Autodesk Inventor part; units mm, degrees
(part 3 of 4)
sketch "Эскиз41" plane through (1.5, 0, 0) normal (1, 0, 0) x (0, 0, -1)
  circle A0 centre (383.6, 368.9) radius 1.625 projected
  circle A1 centre (-13.6, 369) radius 1.625 projected
  circle A2 centre (383.6, 1.1) radius 1.625 projected
  circle A3 centre (-13.6, 1.1) radius 1.625 projected
  circle A4 centre (379.0468, 185.0848) radius 1.625 projected
  circle A5 centre (-9.0468, 185.0848) radius 1.625 projected
  circle A6 centre (379, 228) radius 1.625 projected
  circle A7 centre (-9, 228) radius 1.625 projected
  circle A8 centre (316, 368) radius 1.625 projected
  circle A9 centre (299, 228) radius 1.625 projected
  circle A10 centre (54, 228) radius 1.625 projected
  circle A11 centre (71, 142) radius 1.625 projected
  circle A12 centre (71, 2.0002) radius 1.625 projected
  circle A13 centre (54, 2.0002) radius 1.625 projected
  circle A14 centre (71, 368) radius 1.625 projected
  circle A15 centre (71, 228) radius 1.625 projected
  circle A16 centre (316, 142) radius 1.625 projected
  circle A17 centre (316, 228) radius 1.625 projected
  circle A18 centre (183.175, 129.0059) radius 1.85 projected
  circle A19 centre (299, 368) radius 1.625 projected
  circle A20 centre (316, 2.0002) radius 1.625 projected
  circle A21 centre (54, 142) radius 1.625 projected
  circle A22 centre (54, 368) radius 1.625 projected
  circle A23 centre (299, 2.0002) radius 1.625 projected
  circle A24 centre (299, 142) radius 1.625 projected
  arc A25 (185, 193.309) -> (185, 192.7028) centre (183.175, 193.0059) ccw projected
  line L0 (185, 193.309) -> (185, 192.7028) projected
  line L1 (14.5, 247.5001) -> (35, 247.5001) projected
  arc A26 (38, 244.5001) -> (35, 247.5001) centre (35, 244.5001) ccw projected
  line L2 (38, 244.5001) -> (38, 185.5001) projected
  arc A27 (35, 182.5001) -> (38, 185.5001) centre (35, 185.5001) ccw projected
  line L3 (35, 182.5001) -> (14.5, 182.5001) projected
  arc A28 (11.5, 185.5001) -> (14.5, 182.5001) centre (14.5, 185.5001) ccw projected
  line L4 (11.5, 185.5001) -> (11.5, 244.5001) projected
  arc A29 (14.5, 247.5001) -> (11.5, 244.5001) centre (14.5, 244.5001) ccw projected
  line L5 (358.5, 244.5001) -> (358.5, 185.5001) projected
  arc A30 (355.5, 182.5001) -> (358.5, 185.5001) centre (355.5, 185.5001) ccw projected
  line L6 (355.5, 182.5001) -> (335, 182.5001) projected
  arc A31 (332, 185.5001) -> (335, 182.5001) centre (335, 185.5001) ccw projected
  line L7 (332, 185.5001) -> (332, 244.5001) projected
  arc A32 (335, 247.5001) -> (332, 244.5001) centre (335, 244.5001) ccw projected
  line L8 (335, 247.5001) -> (355.5, 247.5001) projected
  arc A33 (358.5, 244.5001) -> (355.5, 247.5001) centre (355.5, 244.5001) ccw projected
  line L9 (98.825, 226.3849) -> (98.825, 137.3849) projected
  arc A34 (95.825, 134.3849) -> (98.825, 137.3849) centre (95.825, 137.3849) ccw projected
  line L10 (95.825, 134.3849) -> (87.825, 134.3849) projected
  arc A35 (84.825, 137.3849) -> (87.825, 134.3849) centre (87.825, 137.3849) ccw projected
  line L11 (84.825, 137.3849) -> (84.825, 226.3849) projected
  arc A36 (87.825, 229.3849) -> (84.825, 226.3849) centre (87.825, 226.3849) ccw projected
  line L12 (87.825, 229.3849) -> (95.825, 229.3849) projected
  arc A37 (98.825, 226.3849) -> (95.825, 229.3849) centre (95.825, 226.3849) ccw projected
  circle A38 centre (124.375, 129.0059) radius 2 projected
  circle A39 centre (124.375, 193.0059) radius 2 projected
  circle A40 centre (217.25, 312.9941) radius 2.1 projected
  circle A41 centre (152.75, 57.0059) radius 2.1 projected
  circle A42 centre (152.75, 118.0059) radius 2.1 projected
  circle A43 centre (152.75, 312.9941) radius 2.1 projected
  circle A44 centre (217.25, 251.9941) radius 2.1 projected
  circle A45 centre (217.25, 57.0059) radius 2.1 projected
  circle A46 centre (217.25, 118.0059) radius 2.1 projected
  circle A47 centre (152.75, 251.9941) radius 2.1 projected
  line L13 (165, 44) -> (165, 8) projected
  arc A48 (162, 5) -> (165, 8) centre (162, 8) ccw projected
  line L14 (162, 5) -> (96, 5) projected
  arc A49 (93, 8) -> (96, 5) centre (96, 8) ccw projected
  line L15 (93, 8) -> (93, 44) projected
  arc A50 (96, 47) -> (93, 44) centre (96, 44) ccw projected
  line L16 (96, 47) -> (162, 47) projected
  arc A51 (165, 44) -> (162, 47) centre (162, 44) ccw projected
  circle A52 centre (319.1128, 165.0002) radius 2.1 projected
  circle A53 centre (287, 56.343) radius 2.1 projected
  circle A54 centre (50.8872, 165.0002) radius 2.1 projected
  circle A55 centre (173.9908, 56.343) radius 2.1 projected
  circle A56 centre (135.25, 60) radius 2.1 projected
  circle A57 centre (103, 60) radius 2.1 projected
  line L17 (226.25, 270.0041) -> (226.25, 298.657) projected
  arc A58 (228.25, 300.657) -> (226.25, 298.657) centre (228.25, 298.657) ccw projected
  line L18 (228.25, 300.657) -> (268.3252, 300.657) projected
  arc A59 (269.4885, 297.03) -> (268.3252, 300.657) centre (268.3252, 298.657) ccw projected
  line L19 (269.4885, 297.03) -> (229.4132, 268.3772) projected
  arc A60 (226.25, 270.0041) -> (229.4132, 268.3772) centre (228.25, 270.0041) ccw projected
  arc A61 (235.9248, 170.343) -> (234.7615, 166.7161) centre (235.9248, 168.343) ccw projected
  line L20 (235.9248, 170.343) -> (276, 170.343) projected
  arc A62 (278, 168.343) -> (276, 170.343) centre (276, 168.343) ccw projected
  line L21 (278, 168.343) -> (278, 139.6902) projected
  arc A63 (274.8368, 138.0633) -> (278, 139.6902) centre (276, 139.6902) ccw projected
  line L22 (274.8368, 138.0633) -> (234.7615, 166.7161) projected
  arc A64 (94, 106.343) -> (92, 104.343) centre (94, 104.343) ccw projected
  line L23 (94, 106.343) -> (134.0752, 106.343) projected
  arc A65 (135.2385, 102.7161) -> (134.0752, 106.343) centre (134.0752, 104.343) ccw projected
  line L24 (135.2385, 102.7161) -> (95.1632, 74.0633) projected
  arc A66 (92, 75.6902) -> (95.1632, 74.0633) centre (94, 75.6902) ccw projected
  line L25 (92, 75.6902) -> (92, 104.343) projected
  arc A67 (92, 265.657) -> (94, 263.657) centre (94, 265.657) ccw projected
  line L26 (92, 265.657) -> (92, 294.3098) projected
  arc A68 (95.1632, 295.9367) -> (92, 294.3098) centre (94, 294.3098) ccw projected
  line L27 (95.1632, 295.9367) -> (135.2385, 267.2839) projected
  arc A69 (134.0752, 263.657) -> (135.2385, 267.2839) centre (134.0752, 265.657) ccw projected
  line L28 (134.0752, 263.657) -> (94, 263.657) projected
  arc A70 (130.725, 206.0059) -> (132.725, 204.0059) centre (132.725, 206.0059) ccw projected
  line L29 (130.725, 206.0059) -> (130.725, 234.2716) projected
  arc A71 (133.9769, 235.8314) -> (130.725, 234.2716) centre (132.725, 234.2716) ccw projected
  line L30 (133.9769, 235.8314) -> (169.1945, 207.5656) projected
  arc A72 (167.9426, 204.0059) -> (169.1945, 207.5656) centre (167.9426, 206.0059) ccw projected
  line L31 (167.9426, 204.0059) -> (132.725, 204.0059) projected
  arc A73 (226.25, 71.343) -> (228.25, 69.343) centre (228.25, 71.343) ccw projected
  line L32 (226.25, 71.343) -> (226.25, 99.9959) projected
  arc A74 (229.4132, 101.6228) -> (226.25, 99.9959) centre (228.25, 99.9959) ccw projected
  line L33 (229.4132, 101.6228) -> (269.4885, 72.97) projected
  arc A75 (268.3252, 69.343) -> (269.4885, 72.97) centre (268.3252, 71.343) ccw projected
  line L34 (268.3252, 69.343) -> (228.25, 69.343) projected
  arc A76 (226.25, 201.657) -> (228.25, 199.657) centre (228.25, 201.657) ccw projected
  line L35 (226.25, 201.657) -> (226.25, 230.3098) projected
  arc A77 (229.4132, 231.9367) -> (226.25, 230.3098) centre (228.25, 230.3098) ccw projected
  line L36 (229.4132, 231.9367) -> (269.4885, 203.2839) projected
  arc A78 (268.3252, 199.657) -> (269.4885, 203.2839) centre (268.3252, 201.657) ccw projected
  line L37 (268.3252, 199.657) -> (228.25, 199.657) projected
  arc A79 (278, 294.3098) -> (274.8368, 295.9367) centre (276, 294.3098) ccw projected
  line L38 (278, 294.3098) -> (278, 265.657) projected
  arc A80 (276, 263.657) -> (278, 265.657) centre (276, 265.657) ccw projected
  line L39 (276, 263.657) -> (235.9248, 263.657) projected
  arc A81 (234.7615, 267.2839) -> (235.9248, 263.657) centre (235.9248, 265.657) ccw projected
  line L40 (234.7615, 267.2839) -> (274.8368, 295.9367) projected
  arc A82 (226.25, 135.343) -> (228.25, 133.343) centre (228.25, 135.343) ccw projected
  line L41 (226.25, 135.343) -> (226.25, 163.9959) projected
  arc A83 (229.4132, 165.6228) -> (226.25, 163.9959) centre (228.25, 163.9959) ccw projected
  line L42 (229.4132, 165.6228) -> (269.4885, 136.97) projected
  arc A84 (268.3252, 133.343) -> (269.4885, 136.97) centre (268.3252, 135.343) ccw projected
  line L43 (268.3252, 133.343) -> (228.25, 133.343) projected
  arc A85 (143.75, 99.9959) -> (140.5868, 101.6228) centre (141.75, 99.9959) ccw projected
  line L44 (143.75, 99.9959) -> (143.75, 71.343) projected
  arc A86 (141.75, 69.343) -> (143.75, 71.343) centre (141.75, 71.343) ccw projected
  line L45 (141.75, 69.343) -> (101.6748, 69.343) projected
  arc A87 (100.5115, 72.97) -> (101.6748, 69.343) centre (101.6748, 71.343) ccw projected
  line L46 (100.5115, 72.97) -> (140.5868, 101.6228) projected
  arc A88 (143.75, 298.657) -> (141.75, 300.657) centre (141.75, 298.657) ccw projected
  line L47 (143.75, 298.657) -> (143.75, 270.0041) projected
  arc A89 (140.5868, 268.3772) -> (143.75, 270.0041) centre (141.75, 270.0041) ccw projected
  line L48 (140.5868, 268.3772) -> (100.5115, 297.03) projected
  arc A90 (101.6748, 300.657) -> (100.5115, 297.03) centre (101.6748, 298.657) ccw projected
  line L49 (101.6748, 300.657) -> (141.75, 300.657) projected
  line L50 (176.825, 239.0059) -> (176.825, 210.7401) projected
  arc A91 (173.5731, 209.1803) -> (176.825, 210.7401) centre (174.825, 210.7401) ccw projected
  line L51 (173.5731, 209.1803) -> (138.3555, 237.4461) projected
  arc A92 (139.6074, 241.0059) -> (138.3555, 237.4461) centre (139.6074, 239.0059) ccw projected
  line L52 (139.6074, 241.0059) -> (174.825, 241.0059) projected
  arc A93 (176.825, 239.0059) -> (174.825, 241.0059) centre (174.825, 239.0059) ccw projected
  line L53 (278, 104.343) -> (278, 75.6902) projected
  arc A94 (274.8368, 74.0633) -> (278, 75.6902) centre (276, 75.6902) ccw projected
  line L54 (274.8368, 74.0633) -> (234.7615, 102.7161) projected
  arc A95 (235.9248, 106.343) -> (234.7615, 102.7161) centre (235.9248, 104.343) ccw projected
  line L55 (235.9248, 106.343) -> (276, 106.343) projected
  arc A96 (278, 104.343) -> (276, 106.343) centre (276, 104.343) ccw projected
  arc A97 (278, 234.657) -> (276, 236.657) centre (276, 234.657) ccw projected
  line L56 (278, 234.657) -> (278, 206.0041) projected
  arc A98 (274.8368, 204.3772) -> (278, 206.0041) centre (276, 206.0041) ccw projected
  line L57 (274.8368, 204.3772) -> (234.7615, 233.03) projected
  arc A99 (235.9248, 236.657) -> (234.7615, 233.03) centre (235.9248, 234.657) ccw projected
  line L58 (235.9248, 236.657) -> (276, 236.657) projected
  arc A100 (295, 375) -> (292, 372) centre (295, 372) ccw projected
  line L59 (292, 372) -> (292, 323.5966) projected
  arc A101 (289, 320.5966) -> (292, 323.5966) centre (289, 323.5966) ccw projected
  line L60 (289, 320.5966) -> (81, 320.5966) projected
  arc A102 (78, 323.5966) -> (81, 320.5966) centre (81, 323.5966) ccw projected
  line L61 (78, 323.5966) -> (78, 372) projected
  arc A103 (78, 372) -> (75, 375) centre (75, 372) ccw projected
  line L62 (75, 375) -> (-15, 375) projected
  arc A104 (-15, 375) -> (-18, 372) centre (-15, 372) ccw projected
  line L63 (-18, 372) -> (-18, -2) projected
  arc A105 (-18, -2) -> (-15, -5) centre (-15, -2) ccw projected
  line L64 (-15, -5) -> (385, -5) projected
  arc A106 (385, -5) -> (388, -2) centre (385, -2) ccw projected
  line L65 (388, -2) -> (388, 372) projected
  arc A107 (388, 372) -> (385, 375) centre (385, 372) ccw projected
  line L66 (385, 375) -> (295, 375) projected
  line L67 (49, 266.848) -> (-8, 266.848) projected
  arc A108 (-11, 269.848) -> (-8, 266.848) centre (-8, 269.848) ccw projected
  line L68 (-11, 269.848) -> (-11, 367) projected
  arc A109 (-8, 370) -> (-11, 367) centre (-8, 367) ccw projected
  line L69 (-8, 370) -> (-7.7889, 370) projected
  arc A110 (-4.2111, 370) -> (-7.7889, 370) centre (-6, 368.9) ccw projected
  line L70 (-4.2111, 370) -> (37, 370) projected
  arc A111 (40, 367) -> (37, 370) centre (37, 367) ccw projected
  line L71 (40, 367) -> (40, 341.848) projected
  arc A112 (40, 341.848) -> (43, 338.848) centre (43, 341.848) ccw projected
  line L72 (43, 338.848) -> (49, 338.848) projected
  arc A113 (52, 335.848) -> (49, 338.848) centre (49, 335.848) ccw projected
  line L73 (52, 335.848) -> (52, 269.848) projected
  arc A114 (49, 266.848) -> (52, 269.848) centre (49, 269.848) ccw projected
  line L74 (374.2111, 0) -> (333, 0) projected
  arc A115 (330, 3) -> (333, 0) centre (333, 3) ccw projected
  line L75 (330, 3) -> (330, 28.152) projected
  arc A116 (330, 28.152) -> (327, 31.152) centre (327, 28.152) ccw projected
  line L76 (327, 31.152) -> (321, 31.152) projected
  arc A117 (318, 34.152) -> (321, 31.152) centre (321, 34.152) ccw projected
  line L77 (318, 34.152) -> (318, 100.152) projected
  arc A118 (321, 103.152) -> (318, 100.152) centre (321, 100.152) ccw projected
  line L78 (321, 103.152) -> (327, 103.152) projected
  arc A119 (327, 103.152) -> (330, 106.152) centre (327, 106.152) ccw projected
  line L79 (330, 106.152) -> (330, 160) projected
  arc A120 (333, 163) -> (330, 160) centre (333, 160) ccw projected
  line L80 (333, 163) -> (377, 163) projected
  arc A121 (380, 160) -> (377, 163) centre (377, 160) ccw projected
  line L81 (380, 160) -> (380, 3) projected
  arc A122 (377.8605, 0.1261) -> (380, 3) centre (377, 3) ccw projected
  arc A123 (374.2111, 0) -> (377.8605, 0.1261) centre (376, 1.1) ccw projected
  line L82 (-7, 163) -> (37, 163) projected
  arc A124 (40, 160) -> (37, 163) centre (37, 160) ccw projected
  line L83 (40, 160) -> (40, 106.152) projected
  arc A125 (40, 106.152) -> (43, 103.152) centre (43, 106.152) ccw projected
  line L84 (43, 103.152) -> (49, 103.152) projected
  arc A126 (52, 100.152) -> (49, 103.152) centre (49, 100.152) ccw projected
  line L85 (52, 100.152) -> (52, 34.152) projected
  arc A127 (49, 31.152) -> (52, 34.152) centre (49, 34.152) ccw projected
  line L86 (49, 31.152) -> (43, 31.152) projected
  arc A128 (43, 31.152) -> (40, 28.152) centre (43, 28.152) ccw projected
  line L87 (40, 28.152) -> (40, 3) projected
  arc A129 (37, 0) -> (40, 3) centre (37, 3) ccw projected
  line L88 (37, 0) -> (-4.2111, 0) projected
  arc A130 (-7.8605, 0.1261) -> (-4.2111, 0) centre (-6, 1.1) ccw projected
  arc A131 (-10, 3) -> (-7.8605, 0.1261) centre (-7, 3) ccw projected
  line L89 (-10, 3) -> (-10, 160) projected
  arc A132 (-7, 163) -> (-10, 160) centre (-7, 160) ccw projected
  line L90 (377, 266.848) -> (321, 266.848) projected
  arc A133 (318, 269.848) -> (321, 266.848) centre (321, 269.848) ccw projected
  line L91 (318, 269.848) -> (318, 335.848) projected
  arc A134 (321, 338.848) -> (318, 335.848) centre (321, 335.848) ccw projected
  line L92 (321, 338.848) -> (327, 338.848) projected
  arc A135 (327, 338.848) -> (330, 341.848) centre (327, 341.848) ccw projected
  line L93 (330, 341.848) -> (330, 367) projected
  arc A136 (333, 370) -> (330, 367) centre (333, 367) ccw projected
  line L94 (333, 370) -> (374.2111, 370) projected
  arc A137 (377.8605, 369.8739) -> (374.2111, 370) centre (376, 368.9) ccw projected
  arc A138 (380, 367) -> (377.8605, 369.8739) centre (377, 367) ccw projected
  line L95 (380, 367) -> (380, 269.848) projected
  arc A139 (377, 266.848) -> (380, 269.848) centre (377, 269.848) ccw projected
  circle A140 centre (-7, 3) radius 3
  line L96 (-4.2111, 0) -> (-7, 0)
  circle A141 centre (377, 3) radius 3
  line L97 (374.2111, 0) -> (377, 0)
  line L98 (-18, -2) -> (-18, 372) projected
  circle A142 centre (-7, 367) radius 3
  line L99 (-4.2111, 370) -> (-7, 370)
  circle A143 centre (377, 367) radius 3
  line L100 (374.2111, 370) -> (377, 370)
  line L101 (185, -5) -> (185, 9)
  line L102 (-7, 266.848) -> (49, 266.848)
  arc A144 (49, 266.848) -> (52, 269.848) centre (49, 269.848) ccw
  line L103 (52, 269.848) -> (52, 335.848)
  arc A145 (52, 335.848) -> (49, 338.848) centre (49, 335.848) ccw
  line L104 (49, 338.848) -> (43, 338.848)
  arc A146 (40, 341.848) -> (43, 338.848) centre (43, 341.848) ccw
  line L105 (40, 341.848) -> (40, 367)
  arc A147 (40, 367) -> (37, 370) centre (37, 367) ccw
  line L106 (37, 370) -> (-4.2111, 370)
  line L107 (-10, 367) -> (-10, 269.848)
  arc A148 (-10, 269.848) -> (-7, 266.848) centre (-7, 269.848) ccw
  circle A149 centre (-7, 367) radius 3
  line L108 (-4.2111, 370) -> (-7, 370)
  point P0 (0, 0)
  point P1 (377.8605, 0.1261)
  constraints: 24 end point, 10 point on circle, 9 symmetric about line, 5 centre point, 2 coincident, 2 vertical, 1 horizontal, 1 midpoint, 1 vertical alignment, 20 other
extrude "Выдавливание35" add sketch "Эскиз41" against normal blind 1.5 contours L67 A108 L68 A109 L69 A110 L99 A142 L107 A148 | L97 A141 A123 | A140 L96 A130 | A143 L100 A137
sketch "Эскиз42" plane through (1.5, 0, 0) normal (1, 0, 0) x (0, 0, -1)
  circle A0 centre (383.6, 368.9) radius 1.625 projected
  circle A1 centre (-13.6, 369) radius 1.625 projected
  circle A2 centre (383.6, 1.1) radius 1.625 projected
  circle A3 centre (-13.6, 1.1) radius 1.625 projected
  circle A4 centre (379.0468, 185.0848) radius 1.625 projected
  circle A5 centre (-9.0468, 185.0848) radius 1.625 projected
  circle A6 centre (379, 228) radius 1.625 projected
  circle A7 centre (-9, 228) radius 1.625 projected
  circle A8 centre (316, 368) radius 1.625 projected
  circle A9 centre (299, 228) radius 1.625 projected
  circle A10 centre (54, 228) radius 1.625 projected
  circle A11 centre (71, 142) radius 1.625 projected
  circle A12 centre (71, 2.0002) radius 1.625 projected
  circle A13 centre (54, 2.0002) radius 1.625 projected
  circle A14 centre (71, 368) radius 1.625 projected
  circle A15 centre (71, 228) radius 1.625 projected
  circle A16 centre (316, 142) radius 1.625 projected
  circle A17 centre (316, 228) radius 1.625 projected
  circle A18 centre (183.175, 129.0059) radius 1.85 projected
  circle A19 centre (299, 368) radius 1.625 projected
  circle A20 centre (316, 2.0002) radius 1.625 projected
  circle A21 centre (54, 142) radius 1.625 projected
  circle A22 centre (54, 368) radius 1.625 projected
  circle A23 centre (299, 2.0002) radius 1.625 projected
  circle A24 centre (299, 142) radius 1.625 projected
  arc A25 (185, 193.309) -> (185, 192.7028) centre (183.175, 193.0059) ccw projected
  line L0 (185, 193.309) -> (185, 192.7028) projected
  line L1 (14.5, 247.5001) -> (35, 247.5001) projected
  arc A26 (38, 244.5001) -> (35, 247.5001) centre (35, 244.5001) ccw projected
  line L2 (38, 244.5001) -> (38, 185.5001) projected
  arc A27 (35, 182.5001) -> (38, 185.5001) centre (35, 185.5001) ccw projected
  line L3 (35, 182.5001) -> (14.5, 182.5001) projected
  arc A28 (11.5, 185.5001) -> (14.5, 182.5001) centre (14.5, 185.5001) ccw projected
  line L4 (11.5, 185.5001) -> (11.5, 244.5001) projected
  arc A29 (14.5, 247.5001) -> (11.5, 244.5001) centre (14.5, 244.5001) ccw projected
  line L5 (358.5, 244.5001) -> (358.5, 185.5001) projected
  arc A30 (355.5, 182.5001) -> (358.5, 185.5001) centre (355.5, 185.5001) ccw projected
  line L6 (355.5, 182.5001) -> (335, 182.5001) projected
  arc A31 (332, 185.5001) -> (335, 182.5001) centre (335, 185.5001) ccw projected
  line L7 (332, 185.5001) -> (332, 244.5001) projected
  arc A32 (335, 247.5001) -> (332, 244.5001) centre (335, 244.5001) ccw projected
  line L8 (335, 247.5001) -> (355.5, 247.5001) projected
  arc A33 (358.5, 244.5001) -> (355.5, 247.5001) centre (355.5, 244.5001) ccw projected
  line L9 (98.825, 226.3849) -> (98.825, 137.3849) projected
  arc A34 (95.825, 134.3849) -> (98.825, 137.3849) centre (95.825, 137.3849) ccw projected
  line L10 (95.825, 134.3849) -> (87.825, 134.3849) projected
  arc A35 (84.825, 137.3849) -> (87.825, 134.3849) centre (87.825, 137.3849) ccw projected
  line L11 (84.825, 137.3849) -> (84.825, 226.3849) projected
  arc A36 (87.825, 229.3849) -> (84.825, 226.3849) centre (87.825, 226.3849) ccw projected
  line L12 (87.825, 229.3849) -> (95.825, 229.3849) projected
  arc A37 (98.825, 226.3849) -> (95.825, 229.3849) centre (95.825, 226.3849) ccw projected
  circle A38 centre (124.375, 129.0059) radius 2 projected
  circle A39 centre (124.375, 193.0059) radius 2 projected
  circle A40 centre (217.25, 312.9941) radius 2.1 projected
  circle A41 centre (152.75, 57.0059) radius 2.1 projected
  circle A42 centre (152.75, 118.0059) radius 2.1 projected
  circle A43 centre (152.75, 312.9941) radius 2.1 projected
  circle A44 centre (217.25, 251.9941) radius 2.1 projected
  circle A45 centre (217.25, 57.0059) radius 2.1 projected
  circle A46 centre (217.25, 118.0059) radius 2.1 projected
  circle A47 centre (152.75, 251.9941) radius 2.1 projected
  line L13 (165, 44) -> (165, 8) projected
  arc A48 (162, 5) -> (165, 8) centre (162, 8) ccw projected
  line L14 (162, 5) -> (96, 5) projected
  arc A49 (93, 8) -> (96, 5) centre (96, 8) ccw projected
  line L15 (93, 8) -> (93, 44) projected
  arc A50 (96, 47) -> (93, 44) centre (96, 44) ccw projected
  line L16 (96, 47) -> (162, 47) projected
  arc A51 (165, 44) -> (162, 47) centre (162, 44) ccw projected
  circle A52 centre (319.1128, 165.0002) radius 2.1 projected
  circle A53 centre (287, 56.343) radius 2.1 projected
  circle A54 centre (50.8872, 165.0002) radius 2.1 projected
  circle A55 centre (173.9908, 56.343) radius 2.1 projected
  circle A56 centre (135.25, 60) radius 2.1 projected
  circle A57 centre (103, 60) radius 2.1 projected
  line L17 (226.25, 270.0041) -> (226.25, 298.657) projected
  arc A58 (228.25, 300.657) -> (226.25, 298.657) centre (228.25, 298.657) ccw projected
  line L18 (228.25, 300.657) -> (268.3252, 300.657) projected
  arc A59 (269.4885, 297.03) -> (268.3252, 300.657) centre (268.3252, 298.657) ccw projected
  line L19 (269.4885, 297.03) -> (229.4132, 268.3772) projected
  arc A60 (226.25, 270.0041) -> (229.4132, 268.3772) centre (228.25, 270.0041) ccw projected
  arc A61 (235.9248, 170.343) -> (234.7615, 166.7161) centre (235.9248, 168.343) ccw projected
  line L20 (235.9248, 170.343) -> (276, 170.343) projected
  arc A62 (278, 168.343) -> (276, 170.343) centre (276, 168.343) ccw projected
  line L21 (278, 168.343) -> (278, 139.6902) projected
  arc A63 (274.8368, 138.0633) -> (278, 139.6902) centre (276, 139.6902) ccw projected
  line L22 (274.8368, 138.0633) -> (234.7615, 166.7161) projected
  arc A64 (94, 106.343) -> (92, 104.343) centre (94, 104.343) ccw projected
  line L23 (94, 106.343) -> (134.0752, 106.343) projected
  arc A65 (135.2385, 102.7161) -> (134.0752, 106.343) centre (134.0752, 104.343) ccw projected
  line L24 (135.2385, 102.7161) -> (95.1632, 74.0633) projected
  arc A66 (92, 75.6902) -> (95.1632, 74.0633) centre (94, 75.6902) ccw projected
  line L25 (92, 75.6902) -> (92, 104.343) projected
  arc A67 (92, 265.657) -> (94, 263.657) centre (94, 265.657) ccw projected
  line L26 (92, 265.657) -> (92, 294.3098) projected
  arc A68 (95.1632, 295.9367) -> (92, 294.3098) centre (94, 294.3098) ccw projected
  line L27 (95.1632, 295.9367) -> (135.2385, 267.2839) projected
  arc A69 (134.0752, 263.657) -> (135.2385, 267.2839) centre (134.0752, 265.657) ccw projected
  line L28 (134.0752, 263.657) -> (94, 263.657) projected
  arc A70 (130.725, 206.0059) -> (132.725, 204.0059) centre (132.725, 206.0059) ccw projected
  line L29 (130.725, 206.0059) -> (130.725, 234.2716) projected
  arc A71 (133.9769, 235.8314) -> (130.725, 234.2716) centre (132.725, 234.2716) ccw projected
  line L30 (133.9769, 235.8314) -> (169.1945, 207.5656) projected
  arc A72 (167.9426, 204.0059) -> (169.1945, 207.5656) centre (167.9426, 206.0059) ccw projected
  line L31 (167.9426, 204.0059) -> (132.725, 204.0059) projected
  arc A73 (226.25, 71.343) -> (228.25, 69.343) centre (228.25, 71.343) ccw projected
  line L32 (226.25, 71.343) -> (226.25, 99.9959) projected
  arc A74 (229.4132, 101.6228) -> (226.25, 99.9959) centre (228.25, 99.9959) ccw projected
  line L33 (229.4132, 101.6228) -> (269.4885, 72.97) projected
  arc A75 (268.3252, 69.343) -> (269.4885, 72.97) centre (268.3252, 71.343) ccw projected
  line L34 (268.3252, 69.343) -> (228.25, 69.343) projected
  arc A76 (226.25, 201.657) -> (228.25, 199.657) centre (228.25, 201.657) ccw projected
  line L35 (226.25, 201.657) -> (226.25, 230.3098) projected
  arc A77 (229.4132, 231.9367) -> (226.25, 230.3098) centre (228.25, 230.3098) ccw projected
  line L36 (229.4132, 231.9367) -> (269.4885, 203.2839) projected
  arc A78 (268.3252, 199.657) -> (269.4885, 203.2839) centre (268.3252, 201.657) ccw projected
  line L37 (268.3252, 199.657) -> (228.25, 199.657) projected
  arc A79 (278, 294.3098) -> (274.8368, 295.9367) centre (276, 294.3098) ccw projected
  line L38 (278, 294.3098) -> (278, 265.657) projected
  arc A80 (276, 263.657) -> (278, 265.657) centre (276, 265.657) ccw projected
  line L39 (276, 263.657) -> (235.9248, 263.657) projected
  arc A81 (234.7615, 267.2839) -> (235.9248, 263.657) centre (235.9248, 265.657) ccw projected
  line L40 (234.7615, 267.2839) -> (274.8368, 295.9367) projected
  arc A82 (226.25, 135.343) -> (228.25, 133.343) centre (228.25, 135.343) ccw projected
  line L41 (226.25, 135.343) -> (226.25, 163.9959) projected
  arc A83 (229.4132, 165.6228) -> (226.25, 163.9959) centre (228.25, 163.9959) ccw projected
  line L42 (229.4132, 165.6228) -> (269.4885, 136.97) projected
  arc A84 (268.3252, 133.343) -> (269.4885, 136.97) centre (268.3252, 135.343) ccw projected
  line L43 (268.3252, 133.343) -> (228.25, 133.343) projected
  arc A85 (143.75, 99.9959) -> (140.5868, 101.6228) centre (141.75, 99.9959) ccw projected
  line L44 (143.75, 99.9959) -> (143.75, 71.343) projected
  arc A86 (141.75, 69.343) -> (143.75, 71.343) centre (141.75, 71.343) ccw projected
  line L45 (141.75, 69.343) -> (101.6748, 69.343) projected
  arc A87 (100.5115, 72.97) -> (101.6748, 69.343) centre (101.6748, 71.343) ccw projected
  line L46 (100.5115, 72.97) -> (140.5868, 101.6228) projected
  arc A88 (143.75, 298.657) -> (141.75, 300.657) centre (141.75, 298.657) ccw projected
  line L47 (143.75, 298.657) -> (143.75, 270.0041) projected
  arc A89 (140.5868, 268.3772) -> (143.75, 270.0041) centre (141.75, 270.0041) ccw projected
  line L48 (140.5868, 268.3772) -> (100.5115, 297.03) projected
  arc A90 (101.6748, 300.657) -> (100.5115, 297.03) centre (101.6748, 298.657) ccw projected
  line L49 (101.6748, 300.657) -> (141.75, 300.657) projected
  line L50 (176.825, 239.0059) -> (176.825, 210.7401) projected
  arc A91 (173.5731, 209.1803) -> (176.825, 210.7401) centre (174.825, 210.7401) ccw projected
  line L51 (173.5731, 209.1803) -> (138.3555, 237.4461) projected
  arc A92 (139.6074, 241.0059) -> (138.3555, 237.4461) centre (139.6074, 239.0059) ccw projected
  line L52 (139.6074, 241.0059) -> (174.825, 241.0059) projected
  arc A93 (176.825, 239.0059) -> (174.825, 241.0059) centre (174.825, 239.0059) ccw projected
  line L53 (278, 104.343) -> (278, 75.6902) projected
  arc A94 (274.8368, 74.0633) -> (278, 75.6902) centre (276, 75.6902) ccw projected
  line L54 (274.8368, 74.0633) -> (234.7615, 102.7161) projected
  arc A95 (235.9248, 106.343) -> (234.7615, 102.7161) centre (235.9248, 104.343) ccw projected
  line L55 (235.9248, 106.343) -> (276, 106.343) projected
  arc A96 (278, 104.343) -> (276, 106.343) centre (276, 104.343) ccw projected
  arc A97 (278, 234.657) -> (276, 236.657) centre (276, 234.657) ccw projected
  line L56 (278, 234.657) -> (278, 206.0041) projected
  arc A98 (274.8368, 204.3772) -> (278, 206.0041) centre (276, 206.0041) ccw projected
  line L57 (274.8368, 204.3772) -> (234.7615, 233.03) projected
  arc A99 (235.9248, 236.657) -> (234.7615, 233.03) centre (235.9248, 234.657) ccw projected
  line L58 (235.9248, 236.657) -> (276, 236.657) projected
  arc A100 (295, 375) -> (292, 372) centre (295, 372) ccw projected
  line L59 (292, 372) -> (292, 323.5966) projected
  arc A101 (289, 320.5966) -> (292, 323.5966) centre (289, 323.5966) ccw projected
  line L60 (289, 320.5966) -> (81, 320.5966) projected
  arc A102 (78, 323.5966) -> (81, 320.5966) centre (81, 323.5966) ccw projected
  line L61 (78, 323.5966) -> (78, 372) projected
  arc A103 (78, 372) -> (75, 375) centre (75, 372) ccw projected
  line L62 (75, 375) -> (-15, 375) projected
  arc A104 (-15, 375) -> (-18, 372) centre (-15, 372) ccw projected
  line L63 (-18, 372) -> (-18, -2) projected
  arc A105 (-18, -2) -> (-15, -5) centre (-15, -2) ccw projected
  line L64 (-15, -5) -> (385, -5) projected
  arc A106 (385, -5) -> (388, -2) centre (385, -2) ccw projected
  line L65 (388, -2) -> (388, 372) projected
  arc A107 (388, 372) -> (385, 375) centre (385, 372) ccw projected
  line L66 (385, 375) -> (295, 375) projected
  line L67 (49, 266.848) -> (-7, 266.848) projected
  arc A108 (-10, 269.848) -> (-7, 266.848) centre (-7, 269.848) ccw projected
  line L68 (-10, 269.848) -> (-10, 367) projected
  arc A109 (-7, 370) -> (-10, 367) centre (-7, 367) ccw projected
  line L69 (-7, 370) -> (37, 370) projected
  arc A110 (40, 367) -> (37, 370) centre (37, 367) ccw projected
  line L70 (40, 367) -> (40, 341.848) projected
  arc A111 (40, 341.848) -> (43, 338.848) centre (43, 341.848) ccw projected
  line L71 (43, 338.848) -> (49, 338.848) projected
  arc A112 (52, 335.848) -> (49, 338.848) centre (49, 335.848) ccw projected
  line L72 (52, 335.848) -> (52, 269.848) projected
  arc A113 (49, 266.848) -> (52, 269.848) centre (49, 269.848) ccw projected
  line L73 (377, 0) -> (333, 0) projected
  arc A114 (330, 3) -> (333, 0) centre (333, 3) ccw projected
  line L74 (330, 3) -> (330, 28.152) projected
  arc A115 (330, 28.152) -> (327, 31.152) centre (327, 28.152) ccw projected
  line L75 (327, 31.152) -> (321, 31.152) projected
  arc A116 (318, 34.152) -> (321, 31.152) centre (321, 34.152) ccw projected
  line L76 (318, 34.152) -> (318, 100.152) projected
  arc A117 (321, 103.152) -> (318, 100.152) centre (321, 100.152) ccw projected
  line L77 (321, 103.152) -> (327, 103.152) projected
  arc A118 (327, 103.152) -> (330, 106.152) centre (327, 106.152) ccw projected
  line L78 (330, 106.152) -> (330, 160) projected
  arc A119 (333, 163) -> (330, 160) centre (333, 160) ccw projected
  line L79 (333, 163) -> (377, 163) projected
  arc A120 (380, 160) -> (377, 163) centre (377, 160) ccw projected
  line L80 (380, 160) -> (380, 3) projected
  arc A121 (377, 0) -> (380, 3) centre (377, 3) ccw projected
  line L81 (-7, 163) -> (37, 163) projected
  arc A122 (40, 160) -> (37, 163) centre (37, 160) ccw projected
  line L82 (40, 160) -> (40, 106.152) projected
  arc A123 (40, 106.152) -> (43, 103.152) centre (43, 106.152) ccw projected
  line L83 (43, 103.152) -> (49, 103.152) projected
  arc A124 (52, 100.152) -> (49, 103.152) centre (49, 100.152) ccw projected
  line L84 (52, 100.152) -> (52, 34.152) projected
  arc A125 (49, 31.152) -> (52, 34.152) centre (49, 34.152) ccw projected
  line L85 (49, 31.152) -> (43, 31.152) projected
  arc A126 (43, 31.152) -> (40, 28.152) centre (43, 28.152) ccw projected
  line L86 (40, 28.152) -> (40, 3) projected
  arc A127 (37, 0) -> (40, 3) centre (37, 3) ccw projected
  line L87 (37, 0) -> (-7, 0) projected
  arc A128 (-10, 3) -> (-7, 0) centre (-7, 3) ccw projected
  line L88 (-10, 3) -> (-10, 160) projected
  arc A129 (-7, 163) -> (-10, 160) centre (-7, 160) ccw projected
  line L89 (377, 266.848) -> (321, 266.848) projected
  arc A130 (318, 269.848) -> (321, 266.848) centre (321, 269.848) ccw projected
  line L90 (318, 269.848) -> (318, 335.848) projected
  arc A131 (321, 338.848) -> (318, 335.848) centre (321, 335.848) ccw projected
  line L91 (321, 338.848) -> (327, 338.848) projected
  arc A132 (327, 338.848) -> (330, 341.848) centre (327, 341.848) ccw projected
  line L92 (330, 341.848) -> (330, 367) projected
  arc A133 (333, 370) -> (330, 367) centre (333, 367) ccw projected
  line L93 (333, 370) -> (377, 370) projected
  arc A134 (380, 367) -> (377, 370) centre (377, 367) ccw projected
  line L94 (380, 367) -> (380, 269.848) projected
  arc A135 (377, 266.848) -> (380, 269.848) centre (377, 269.848) ccw projected
  line L95 (56, 105.152) -> (56, 29.152)
  line L96 (54, 107.152) -> (40, 107.152)
  line L97 (40, 27.152) -> (54, 27.152)
  line L98 (56, 340.848) -> (56, 264.848)
  line L99 (54, 342.848) -> (40, 342.848)
  line L100 (-8, 262.848) -> (54, 262.848)
  line L101 (-10, 269.848) -> (-10, 264.848)
  arc A136 (56, 340.848) -> (54, 342.848) centre (54, 340.848) ccw
  arc A137 (54, 262.848) -> (56, 264.848) centre (54, 264.848) ccw
  arc A138 (-10, 264.848) -> (-8, 262.848) centre (-8, 264.848) ccw
  arc A139 (56, 105.152) -> (54, 107.152) centre (54, 105.152) ccw
  arc A140 (54, 27.152) -> (56, 29.152) centre (54, 29.152) ccw
  point P0 (0, 0)
  point P1 (56, 107.152)
  point P2 (56, 27.152)
  dimension "d218" = 4
  dimension "d219" = 4
  dimension "d220" = 4
  dimension "d223" = 2
  dimension "d224" = 2
  constraints: 14 end point, 10 point on circle, 10 tangent, 6 point on line, 5 centre point, 4 horizontal, 3 equal radius, 3 vertical
  measures "d218" distance between parallel lines of L84 L95
  measures "d219" distance between parallel lines of L96 L83
  measures "d220" distance from line of L97 L85.start
  measures "d223" radius of A136
  measures "d224" radius of A137
extrude "Выдавливание36" cut sketch "Эскиз42" against normal blind 10 contours A113 L72 A112 L71 A111 L70 L99 A136 L98 A137 L100 A138 L101 A108 L67 | L96 A139 L95 A140 L97 L86 A126 L85 A125 L84 A124 L83 A123 L82
fillet "Сопряжение3" radius 2 3 edges at (0.75, 342.848, -40) (0.75, 107.152, -40) (0.75, 27.152, -40)
sketch "Эскиз43" plane through (1.5, 0, 0) normal (1, 0, 0) x (0, 0, -1)
  arc A0 (42, 27.152) -> (40, 25.152) centre (42, 25.152) ccw projected
  line L0 (40, 25.152) -> (40, 3) projected
  arc A1 (37, 0) -> (40, 3) centre (37, 3) ccw projected
  line L1 (37, 0) -> (-7, 0) projected
  arc A2 (-10, 3) -> (-7, 0) centre (-7, 3) ccw projected
  line L2 (-10, 3) -> (-10, 160) projected
  arc A3 (-7, 163) -> (-10, 160) centre (-7, 160) ccw projected
  line L3 (-7, 163) -> (37, 163) projected
  arc A4 (40, 160) -> (37, 163) centre (37, 160) ccw projected
  line L4 (40, 160) -> (40, 109.152) projected
  arc A5 (40, 109.152) -> (42, 107.152) centre (42, 109.152) ccw projected
  line L5 (42, 107.152) -> (54, 107.152) projected
  arc A6 (56, 105.152) -> (54, 107.152) centre (54, 105.152) ccw projected
  line L6 (56, 105.152) -> (56, 29.152) projected
  arc A7 (54, 27.152) -> (56, 29.152) centre (54, 29.152) ccw projected
  line L7 (54, 27.152) -> (42, 27.152) projected
  circle A8 centre (383.6, 368.9) radius 1.625 projected
  circle A9 centre (-13.6, 369) radius 1.625 projected
  circle A10 centre (383.6, 1.1) radius 1.625 projected
  circle A11 centre (-13.6, 1.1) radius 1.625 projected
  circle A12 centre (379.0468, 185.0848) radius 1.625 projected
  circle A13 centre (-9.0468, 185.0848) radius 1.625 projected
  circle A14 centre (379, 228) radius 1.625 projected
  circle A15 centre (-9, 228) radius 1.625 projected
  circle A16 centre (316, 368) radius 1.625 projected
  circle A17 centre (299, 228) radius 1.625 projected
  circle A18 centre (54, 228) radius 1.625 projected
  circle A19 centre (71, 142) radius 1.625 projected
  circle A20 centre (71, 2.0002) radius 1.625 projected
  circle A21 centre (54, 2.0002) radius 1.625 projected
  circle A22 centre (71, 368) radius 1.625 projected
  circle A23 centre (71, 228) radius 1.625 projected
  circle A24 centre (316, 142) radius 1.625 projected
  circle A25 centre (316, 228) radius 1.625 projected
  circle A26 centre (183.175, 129.0059) radius 1.85 projected
  circle A27 centre (299, 368) radius 1.625 projected
  circle A28 centre (316, 2.0002) radius 1.625 projected
  circle A29 centre (54, 142) radius 1.625 projected
  circle A30 centre (54, 368) radius 1.625 projected
  circle A31 centre (299, 2.0002) radius 1.625 projected
  circle A32 centre (299, 142) radius 1.625 projected
  arc A33 (185, 193.309) -> (185, 192.7028) centre (183.175, 193.0059) ccw projected
  line L8 (185, 193.309) -> (185, 192.7028) projected
  line L9 (14.5, 247.5001) -> (35, 247.5001) projected
  arc A34 (38, 244.5001) -> (35, 247.5001) centre (35, 244.5001) ccw projected
  line L10 (38, 244.5001) -> (38, 185.5001) projected
  arc A35 (35, 182.5001) -> (38, 185.5001) centre (35, 185.5001) ccw projected
  line L11 (35, 182.5001) -> (14.5, 182.5001) projected
  arc A36 (11.5, 185.5001) -> (14.5, 182.5001) centre (14.5, 185.5001) ccw projected
  line L12 (11.5, 185.5001) -> (11.5, 244.5001) projected
  arc A37 (14.5, 247.5001) -> (11.5, 244.5001) centre (14.5, 244.5001) ccw projected
  line L13 (358.5, 244.5001) -> (358.5, 185.5001) projected
  arc A38 (355.5, 182.5001) -> (358.5, 185.5001) centre (355.5, 185.5001) ccw projected
  line L14 (355.5, 182.5001) -> (335, 182.5001) projected
  arc A39 (332, 185.5001) -> (335, 182.5001) centre (335, 185.5001) ccw projected
  line L15 (332, 185.5001) -> (332, 244.5001) projected
  arc A40 (335, 247.5001) -> (332, 244.5001) centre (335, 244.5001) ccw projected
  line L16 (335, 247.5001) -> (355.5, 247.5001) projected
  arc A41 (358.5, 244.5001) -> (355.5, 247.5001) centre (355.5, 244.5001) ccw projected
  line L17 (98.825, 226.3849) -> (98.825, 137.3849) projected
  arc A42 (95.825, 134.3849) -> (98.825, 137.3849) centre (95.825, 137.3849) ccw projected
  line L18 (95.825, 134.3849) -> (87.825, 134.3849) projected
  arc A43 (84.825, 137.3849) -> (87.825, 134.3849) centre (87.825, 137.3849) ccw projected
  line L19 (84.825, 137.3849) -> (84.825, 226.3849) projected
  arc A44 (87.825, 229.3849) -> (84.825, 226.3849) centre (87.825, 226.3849) ccw projected
  line L20 (87.825, 229.3849) -> (95.825, 229.3849) projected
  arc A45 (98.825, 226.3849) -> (95.825, 229.3849) centre (95.825, 226.3849) ccw projected
  circle A46 centre (124.375, 129.0059) radius 2 projected
  circle A47 centre (124.375, 193.0059) radius 2 projected
  circle A48 centre (217.25, 312.9941) radius 2.1 projected
  circle A49 centre (152.75, 57.0059) radius 2.1 projected
  circle A50 centre (152.75, 118.0059) radius 2.1 projected
  circle A51 centre (152.75, 312.9941) radius 2.1 projected
  circle A52 centre (217.25, 251.9941) radius 2.1 projected
  circle A53 centre (217.25, 57.0059) radius 2.1 projected
  circle A54 centre (217.25, 118.0059) radius 2.1 projected
  circle A55 centre (152.75, 251.9941) radius 2.1 projected
  line L21 (165, 44) -> (165, 8) projected
  arc A56 (162, 5) -> (165, 8) centre (162, 8) ccw projected
  line L22 (162, 5) -> (96, 5) projected
  arc A57 (93, 8) -> (96, 5) centre (96, 8) ccw projected
  line L23 (93, 8) -> (93, 44) projected
  arc A58 (96, 47) -> (93, 44) centre (96, 44) ccw projected
  line L24 (96, 47) -> (162, 47) projected
  arc A59 (165, 44) -> (162, 47) centre (162, 44) ccw projected
  circle A60 centre (319.1128, 165.0002) radius 2.1 projected
  circle A61 centre (287, 56.343) radius 2.1 projected
  circle A62 centre (50.8872, 165.0002) radius 2.1 projected
  circle A63 centre (173.9908, 56.343) radius 2.1 projected
  circle A64 centre (135.25, 60) radius 2.1 projected
  circle A65 centre (103, 60) radius 2.1 projected
  line L25 (226.25, 270.0041) -> (226.25, 298.657) projected
  arc A66 (228.25, 300.657) -> (226.25, 298.657) centre (228.25, 298.657) ccw projected
  line L26 (228.25, 300.657) -> (268.3252, 300.657) projected
  arc A67 (269.4885, 297.03) -> (268.3252, 300.657) centre (268.3252, 298.657) ccw projected
  line L27 (269.4885, 297.03) -> (229.4132, 268.3772) projected
  arc A68 (226.25, 270.0041) -> (229.4132, 268.3772) centre (228.25, 270.0041) ccw projected
  arc A69 (235.9248, 170.343) -> (234.7615, 166.7161) centre (235.9248, 168.343) ccw projected
  line L28 (235.9248, 170.343) -> (276, 170.343) projected
  arc A70 (278, 168.343) -> (276, 170.343) centre (276, 168.343) ccw projected
  line L29 (278, 168.343) -> (278, 139.6902) projected
  arc A71 (274.8368, 138.0633) -> (278, 139.6902) centre (276, 139.6902) ccw projected
  line L30 (274.8368, 138.0633) -> (234.7615, 166.7161) projected
  arc A72 (94, 106.343) -> (92, 104.343) centre (94, 104.343) ccw projected
  line L31 (94, 106.343) -> (134.0752, 106.343) projected
  arc A73 (135.2385, 102.7161) -> (134.0752, 106.343) centre (134.0752, 104.343) ccw projected
  line L32 (135.2385, 102.7161) -> (95.1632, 74.0633) projected
  arc A74 (92, 75.6902) -> (95.1632, 74.0633) centre (94, 75.6902) ccw projected
  line L33 (92, 75.6902) -> (92, 104.343) projected
  arc A75 (92, 265.657) -> (94, 263.657) centre (94, 265.657) ccw projected
  line L34 (92, 265.657) -> (92, 294.3098) projected
  arc A76 (95.1632, 295.9367) -> (92, 294.3098) centre (94, 294.3098) ccw projected
  line L35 (95.1632, 295.9367) -> (135.2385, 267.2839) projected
  arc A77 (134.0752, 263.657) -> (135.2385, 267.2839) centre (134.0752, 265.657) ccw projected
  line L36 (134.0752, 263.657) -> (94, 263.657) projected
  arc A78 (130.725, 206.0059) -> (132.725, 204.0059) centre (132.725, 206.0059) ccw projected
  line L37 (130.725, 206.0059) -> (130.725, 234.2716) projected
  arc A79 (133.9769, 235.8314) -> (130.725, 234.2716) centre (132.725, 234.2716) ccw projected
  line L38 (133.9769, 235.8314) -> (169.1945, 207.5656) projected
  arc A80 (167.9426, 204.0059) -> (169.1945, 207.5656) centre (167.9426, 206.0059) ccw projected
  line L39 (167.9426, 204.0059) -> (132.725, 204.0059) projected
  arc A81 (226.25, 71.343) -> (228.25, 69.343) centre (228.25, 71.343) ccw projected
  line L40 (226.25, 71.343) -> (226.25, 99.9959) projected
  arc A82 (229.4132, 101.6228) -> (226.25, 99.9959) centre (228.25, 99.9959) ccw projected
  line L41 (229.4132, 101.6228) -> (269.4885, 72.97) projected
  arc A83 (268.3252, 69.343) -> (269.4885, 72.97) centre (268.3252, 71.343) ccw projected
  line L42 (268.3252, 69.343) -> (228.25, 69.343) projected
  arc A84 (226.25, 201.657) -> (228.25, 199.657) centre (228.25, 201.657) ccw projected
  line L43 (226.25, 201.657) -> (226.25, 230.3098) projected
  arc A85 (229.4132, 231.9367) -> (226.25, 230.3098) centre (228.25, 230.3098) ccw projected
  line L44 (229.4132, 231.9367) -> (269.4885, 203.2839) projected
  arc A86 (268.3252, 199.657) -> (269.4885, 203.2839) centre (268.3252, 201.657) ccw projected
  line L45 (268.3252, 199.657) -> (228.25, 199.657) projected
  arc A87 (278, 294.3098) -> (274.8368, 295.9367) centre (276, 294.3098) ccw projected
  line L46 (278, 294.3098) -> (278, 265.657) projected
  arc A88 (276, 263.657) -> (278, 265.657) centre (276, 265.657) ccw projected
  line L47 (276, 263.657) -> (235.9248, 263.657) projected
  arc A89 (234.7615, 267.2839) -> (235.9248, 263.657) centre (235.9248, 265.657) ccw projected
  line L48 (234.7615, 267.2839) -> (274.8368, 295.9367) projected
  arc A90 (226.25, 135.343) -> (228.25, 133.343) centre (228.25, 135.343) ccw projected
  line L49 (226.25, 135.343) -> (226.25, 163.9959) projected
  arc A91 (229.4132, 165.6228) -> (226.25, 163.9959) centre (228.25, 163.9959) ccw projected
  line L50 (229.4132, 165.6228) -> (269.4885, 136.97) projected
  arc A92 (268.3252, 133.343) -> (269.4885, 136.97) centre (268.3252, 135.343) ccw projected
  line L51 (268.3252, 133.343) -> (228.25, 133.343) projected
  arc A93 (143.75, 99.9959) -> (140.5868, 101.6228) centre (141.75, 99.9959) ccw projected
  line L52 (143.75, 99.9959) -> (143.75, 71.343) projected
  arc A94 (141.75, 69.343) -> (143.75, 71.343) centre (141.75, 71.343) ccw projected
  line L53 (141.75, 69.343) -> (101.6748, 69.343) projected
  arc A95 (100.5115, 72.97) -> (101.6748, 69.343) centre (101.6748, 71.343) ccw projected
  line L54 (100.5115, 72.97) -> (140.5868, 101.6228) projected
  arc A96 (143.75, 298.657) -> (141.75, 300.657) centre (141.75, 298.657) ccw projected
  line L55 (143.75, 298.657) -> (143.75, 270.0041) projected
  arc A97 (140.5868, 268.3772) -> (143.75, 270.0041) centre (141.75, 270.0041) ccw projected
  line L56 (140.5868, 268.3772) -> (100.5115, 297.03) projected
  arc A98 (101.6748, 300.657) -> (100.5115, 297.03) centre (101.6748, 298.657) ccw projected
  line L57 (101.6748, 300.657) -> (141.75, 300.657) projected
  line L58 (176.825, 239.0059) -> (176.825, 210.7401) projected
  arc A99 (173.5731, 209.1803) -> (176.825, 210.7401) centre (174.825, 210.7401) ccw projected
  line L59 (173.5731, 209.1803) -> (138.3555, 237.4461) projected
  arc A100 (139.6074, 241.0059) -> (138.3555, 237.4461) centre (139.6074, 239.0059) ccw projected
  line L60 (139.6074, 241.0059) -> (174.825, 241.0059) projected
  arc A101 (176.825, 239.0059) -> (174.825, 241.0059) centre (174.825, 239.0059) ccw projected
  line L61 (278, 104.343) -> (278, 75.6902) projected
  arc A102 (274.8368, 74.0633) -> (278, 75.6902) centre (276, 75.6902) ccw projected
  line L62 (274.8368, 74.0633) -> (234.7615, 102.7161) projected
  arc A103 (235.9248, 106.343) -> (234.7615, 102.7161) centre (235.9248, 104.343) ccw projected
  line L63 (235.9248, 106.343) -> (276, 106.343) projected
  arc A104 (278, 104.343) -> (276, 106.343) centre (276, 104.343) ccw projected
  arc A105 (278, 234.657) -> (276, 236.657) centre (276, 234.657) ccw projected
  line L64 (278, 234.657) -> (278, 206.0041) projected
  arc A106 (274.8368, 204.3772) -> (278, 206.0041) centre (276, 206.0041) ccw projected
  line L65 (274.8368, 204.3772) -> (234.7615, 233.03) projected
  arc A107 (235.9248, 236.657) -> (234.7615, 233.03) centre (235.9248, 234.657) ccw projected
  line L66 (235.9248, 236.657) -> (276, 236.657) projected
  arc A108 (295, 375) -> (292, 372) centre (295, 372) ccw projected
  line L67 (292, 372) -> (292, 323.5966) projected
  arc A109 (289, 320.5966) -> (292, 323.5966) centre (289, 323.5966) ccw projected
  line L68 (289, 320.5966) -> (81, 320.5966) projected
  arc A110 (78, 323.5966) -> (81, 320.5966) centre (81, 323.5966) ccw projected
  line L69 (78, 323.5966) -> (78, 372) projected
  arc A111 (78, 372) -> (75, 375) centre (75, 372) ccw projected
  line L70 (75, 375) -> (-15, 375) projected
  arc A112 (-15, 375) -> (-18, 372) centre (-15, 372) ccw projected
  line L71 (-18, 372) -> (-18, -2) projected
  arc A113 (-18, -2) -> (-15, -5) centre (-15, -2) ccw projected
  line L72 (-15, -5) -> (385, -5) projected
  arc A114 (385, -5) -> (388, -2) centre (385, -2) ccw projected
  line L73 (388, -2) -> (388, 372) projected
  arc A115 (388, 372) -> (385, 375) centre (385, 372) ccw projected
  line L74 (385, 375) -> (295, 375) projected
  arc A116 (40, 344.848) -> (42, 342.848) centre (42, 344.848) ccw projected
  line L75 (42, 342.848) -> (54, 342.848) projected
  arc A117 (56, 340.848) -> (54, 342.848) centre (54, 340.848) ccw projected
  line L76 (56, 340.848) -> (56, 264.848) projected
  arc A118 (54, 262.848) -> (56, 264.848) centre (54, 264.848) ccw projected
  line L77 (54, 262.848) -> (-8, 262.848) projected
  arc A119 (-10, 264.848) -> (-8, 262.848) centre (-8, 264.848) ccw projected
  line L78 (-10, 264.848) -> (-10, 367) projected
  arc A120 (-7, 370) -> (-10, 367) centre (-7, 367) ccw projected
  line L79 (-7, 370) -> (37, 370) projected
  arc A121 (40, 367) -> (37, 370) centre (37, 367) ccw projected
  line L80 (40, 367) -> (40, 344.848) projected
  line L81 (377, 0) -> (333, 0) projected
  arc A122 (330, 3) -> (333, 0) centre (333, 3) ccw projected
  line L82 (330, 3) -> (330, 28.152) projected
  arc A123 (330, 28.152) -> (327, 31.152) centre (327, 28.152) ccw projected
  line L83 (327, 31.152) -> (321, 31.152) projected
  arc A124 (318, 34.152) -> (321, 31.152) centre (321, 34.152) ccw projected
  line L84 (318, 34.152) -> (318, 100.152) projected
  arc A125 (321, 103.152) -> (318, 100.152) centre (321, 100.152) ccw projected
  line L85 (321, 103.152) -> (327, 103.152) projected
  arc A126 (327, 103.152) -> (330, 106.152) centre (327, 106.152) ccw projected
  line L86 (330, 106.152) -> (330, 160) projected
  arc A127 (333, 163) -> (330, 160) centre (333, 160) ccw projected
  line L87 (333, 163) -> (377, 163) projected
  arc A128 (380, 160) -> (377, 163) centre (377, 160) ccw projected
  line L88 (380, 160) -> (380, 3) projected
  arc A129 (377, 0) -> (380, 3) centre (377, 3) ccw projected
  line L89 (377, 266.848) -> (321, 266.848) projected
  arc A130 (318, 269.848) -> (321, 266.848) centre (321, 269.848) ccw projected
  line L90 (318, 269.848) -> (318, 335.848) projected
  arc A131 (321, 338.848) -> (318, 335.848) centre (321, 335.848) ccw projected
  line L91 (321, 338.848) -> (327, 338.848) projected
  arc A132 (327, 338.848) -> (330, 341.848) centre (327, 341.848) ccw projected
  line L92 (330, 341.848) -> (330, 367) projected
  arc A133 (333, 370) -> (330, 367) centre (333, 367) ccw projected
  line L93 (333, 370) -> (377, 370) projected
  arc A134 (380, 367) -> (377, 370) centre (377, 367) ccw projected
  line L94 (380, 367) -> (380, 269.848) projected
  arc A135 (377, 266.848) -> (380, 269.848) centre (377, 269.848) ccw projected
  line L95 (386.5, 372) -> (386.5, -2)
  arc A136 (385, -3.5) -> (386.5, -2) centre (385, -2) ccw
  line L96 (385, -3.5) -> (-15, -3.5)
  arc A137 (-16.5, -2) -> (-15, -3.5) centre (-15, -2) ccw
  line L97 (-16.5, -2) -> (-16.5, 372)
  arc A138 (-15, 373.5) -> (-16.5, 372) centre (-15, 372) ccw
  line L98 (-15, 373.5) -> (75, 373.5)
  arc A139 (76.5, 372) -> (75, 373.5) centre (75, 372) ccw
  line L99 (76.5, 372) -> (76.5, 323.5966)
  arc A140 (76.5, 323.5966) -> (81, 319.0966) centre (81, 323.5966) ccw
  line L100 (81, 319.0966) -> (289, 319.0966)
  arc A141 (289, 319.0966) -> (293.5, 323.5966) centre (289, 323.5966) ccw
  line L101 (293.5, 323.5966) -> (293.5, 372)
  arc A142 (295, 373.5) -> (293.5, 372) centre (295, 372) ccw
  line L102 (295, 373.5) -> (385, 373.5)
  arc A143 (386.5, 372) -> (385, 373.5) centre (385, 372) ccw
  line L103 (306.5, -52.2397) -> (306.5, 178.2463)
  line L104 (305.75, -52.2397) -> (305.75, 178.2463)
  line L105 (314.25, -52.2397) -> (314.25, 178.2463)
  circle A144 centre (316, 2.0002) radius 1.625
  circle A145 centre (316, 142) radius 1.625
  circle A146 centre (316, 368) radius 1.625
  circle A147 centre (299, 368) radius 1.625
  circle A148 centre (299, 228) radius 1.625
  circle A149 centre (299, 142) radius 1.625
  circle A150 centre (299, 2.0002) radius 1.625
  circle A151 centre (314.25, 2.0002) radius 1.625
  circle A152 centre (314.25, 142) radius 1.625
  circle A153 centre (314.25, 368) radius 1.625
  circle A154 centre (297.25, 368) radius 1.625
  circle A155 centre (297.25, 228) radius 1.625
  circle A156 centre (297.25, 142) radius 1.625
  circle A157 centre (297.25, 2.0002) radius 1.625
  circle A158 centre (316, 228) radius 1.625 projected
  circle A159 centre (316, 228) radius 1.625
  circle A160 centre (314.25, 228) radius 1.625
  point P0 (0, 0)
  point P1 (298.125, 366.6307)
  point P2 (298.125, 369.3693)
  point P3 (315.125, 366.6307)
  point P4 (315.125, 369.3693)
  point P5 (298.125, 226.6307)
  point P6 (298.125, 229.3693)
  point P7 (315.125, 226.6307)
  point P8 (315.125, 229.3693)
  point P9 (298.125, 140.6307)
  point P10 (298.125, 143.3693)
  dimension "d226" = 1.5
  dimension "d227" = 80
  dimension "d228" = 0.75
  dimension "d229" = 8.5
  constraints: 24 centre point, 22 end point, 16 point on circle, 8 coincident, 8 concentric, 2 parallel, 1 point on line, 1 vertical, 15 other
  measures "d226" distance between parallel lines of L73 L95
  measures "d227" distance between parallel lines of L95 L103
  measures "d228" distance between parallel lines of L103 L104
  measures "d229" distance between parallel lines of L104 L105
extrude "Выдавливание37" cut sketch "Эскиз43" against normal blind 10 contours A16 A153 | A17 A155 | A152 A24 | A24 A152 L105 | L105 A152 | A25 A160 | A27 A154 | A151 A28 | A28 A151 L105 | L105 A151 | A157 A31 | A31 A157 | A32 A156 picked at (313.2269, 367.8123) picked at (296.2269, 227.8123) picked at (314.8817, 142) picked at (313.2269, 227.8123) picked at (296.2269, 367.8123) picked at (314.8817, 2.0002) picked at (297.8817, 2.0002) picked at (296.2269, 2.1879) picked at (296.2269, 141.8123)